Autodesk Fusion 360 part; units mm, degrees
note: some values were not read from the file. Set by a fixed rule: which sketch regions a step uses.
(part 2 of 4)
  spline S338 degree 3 poles (2.6737, -46.2166) (0.624, -45.5094) (-0.7902, -43.8549) (-1.106, -41.9528) (-1.287, -40.8624) (-1.1003, -39.6959) (-0.5192, -38.6497) knots 0 0 0 0 0.618555 0.618555 0.618555 0.973163 0.973163 0.973163 0.973163
  spline S339 degree 3 poles (-0.5192, -38.6497) (-0.9554, -37.9197) (-1.2418, -37.1573) (-1.2576, -36.3503) (-1.2716, -35.6348) (-1.0747, -34.9439) (-0.7598, -34.2709) knots 0.006673 0.006673 0.006673 0.006673 0.533212 0.533212 0.533212 1 1 1 1
  spline S340 degree 3 poles (-0.7598, -34.2709) (0.1145, -32.4027) (1.9335, -31.179) (4.0147, -30.9406) knots 0 0 0 0 0.893312 0.893312 0.893312 0.893312
  spline S341 degree 3 poles (4.0147, -30.9406) (3.9761, -30.3012) (3.9008, -29.105) (3.8396, -28.1591) knots 0.081568 0.081568 0.081568 0.081568 1 1 1 1
  spline S342 degree 3 poles (3.8396, -28.1591) (3.6928, -25.8896) (3.7601, -22.8302) (4.0082, -20.7539) knots 0 0 0 0 1 1 1 1
  spline S343 degree 3 poles (4.0082, -20.7539) (4.7062, -14.9126) (7.125, -9.921) (11.1287, -6.1499) knots 0 0 0 0 1 1 1 1
  constraint coincident L48.end L50
  constraint coincident L49.start S307
  constraint coincident L49.end S308
extrude "Extrude1" add sketch "Sketch1" against normal blind 2 contours S0 L0 L1 S1 S2 L2 L3 S3 S4 S5 S6 S7 S8 S9 S10 S11 S12 S13 S14 S15 S16 L4 L5 S17 S18 S19 L6 L7 S20 S21 S22 S23 S24 S25 L8 L9 S26 S27 L10 L11 S28 S29 S30 S31 S32 S33 S34 S35 S36 S37 S38 S39 S40 L12 L13 S41 S42 S43 S44 S45 S150 L24 L25 S151 S152 L26 L27 S153 S154 S155 S156 S157 S158 S159 S160 S161 S162 S163 S164 S165 S166 L28 L29 S167 S168 S169 L30 L31 S170 S171 S172 S173 S174 S175 L32 L33 S176 S177 L34 L35 S178 S179 S180 S181 S182 S183 S184 S185 S186 S187 S188 S189 S190 L36 L37 S191 S192 S193 S194 S195 | S46 S47 S48 S49 S50 S51 S52 S53 S54 S55 S56 S57 S58 S59 S60 S61 S62 S63 L14 L15 S64 S65 S66 S67 S68 S69 S70 S71 S72 S73 S74 S75 S76 S77 S196 S197 S198 S199 S200 S201 S202 S203 S204 S205 S206 S207 S208 S209 S210 S211 S212 S213 L38 L39 S214 S215 S216 S217 S218 S219 S220 S221 S222 S223 S224 S225 S226 S227 | S78 S79 S80 S81 S82 S83 S84 S85 S86 S87 S88 S89 S90 S91 S92 S93 S94 S95 S96 S97 S98 S99 S100 S101 S102 S103 S104 S105 S106 S107 S228 S229 S230 S231 S232 S233 S234 S235 S236 S237 S238 S239 S240 S241 S242 S243 S244 S245 S246 S247 S248 S249 S250 S251 S252 S253 S254 S255 S256 S257 | S108 S109 S110 S111 S112 S113 S114 S115 S116 L16 L17 S117 S118 S119 L18 L19 S120 S121 S122 S123 S124 S125 S126 S127 S128 S129 S130 S258 S259 S260 S261 S262 S263 S264 S265 S266 L40 L41 S267 S268 S269 L42 L43 S270 S271 S272 S273 S274 S275 S276 S277 S278 S279 S280 | S131 S132 S133 S134 S135 S136 S137 S138 S139 S140 S141 L20 L21 S142 S143 S144 S145 S146 L22 L23 S147 S148 S149 S281 S282 S283 S284 S285 S286 S287 S288 S289 S290 S291 L44 L45 S292 S293 S294 S295 S296 L46 L47 S297 S298 S299 | L49 S300 S301 S302 S303 S304 S305 S306 S307 S308 L50 L51 S309 S310 S311 S312 S313 L52 S314 S315 L53 L54 S316 S317 S318 S319 S320 S321 S322 S323 S324 S325 S326 S327 S328 S329 S330 S331 L55 S332 S333 S334 S335 S336 S337 S338 S339 S340 S341 S342 S343 makes body 1
extrude "Extrude2" add sketch "Sketch1" along normal blind 5 contours S46 S47 S48 S49 S50 S51 S52 S53 S54 S55 S56 S57 S58 S59 S60 S61 S62 S63 L14 L15 S64 S65 S66 S67 S68 S69 S70 S71 S72 S73 S74 S75 S76 S77 S196 S197 S198 S199 S200 S201 S202 S203 S204 S205 S206 S207 S208 S209 S210 S211 S212 S213 L38 L39 S214 S215 S216 S217 S218 S219 S220 S221 S222 S223 S224 S225 S226 S227 | S78 S79 S80 S81 S82 S83 S84 S85 S86 S87 S88 S89 S90 S91 S92 S93 S94 S95 S96 S97 S98 S99 S100 S101 S102 S103 S104 S105 S106 S107 S228 S229 S230 S231 S232 S233 S234 S235 S236 S237 S238 S239 S240 S241 S242 S243 S244 S245 S246 S247 S248 S249 S250 S251 S252 S253 S254 S255 S256 S257 | S108 S109 S110 S111 S112 S113 S114 S115 S116 L16 L17 S117 S118 S119 L18 L19 S120 S121 S122 S123 S124 S125 S126 S127 S128 S129 S130 S258 S259 S260 S261 S262 S263 S264 S265 S266 L40 L41 S267 S268 S269 L42 L43 S270 S271 S272 S273 S274 S275 S276 S277 S278 S279 S280 | S131 S132 S133 S134 S135 S136 S137 S138 S139 S140 S141 L20 L21 S142 S143 S144 S145 S146 L22 L23 S147 S148 S149 S281 S282 S283 S284 S285 S286 S287 S288 S289 S290 S291 L44 L45 S292 S293 S294 S295 S296 L46 L47 S297 S298 S299 bodies 1
extrude "Extrude3" add sketch "Sketch1" along normal blind 10 contours L49 S300 S301 S302 S303 S304 S305 S306 S307 S308 L50 L51 S309 S310 S311 S312 S313 L52 S314 S315 L53 L54 S316 S317 S318 S319 S320 S321 S322 S323 S324 S325 S326 S327 S328 S329 S330 S331 L55 S332 S333 S334 S335 S336 S337 S338 S339 S340 S341 S342 S343 bodies 1
extrude "Extrude4" add sketch "Sketch1" against normal blind 2 separate body contours S0 L0 L1 S1 S2 L2 L3 S3 S4 S5 S6 S7 S8 S9 S10 S11 S12 S13 S14 S15 S16 L4 L5 S17 S18 S19 L6 L7 S20 S21 S22 S23 S24 S25 L8 L9 S26 S27 L10 L11 S28 S29 S30 S31 S32 S33 S34 S35 S36 S37 S38 S39 S40 L12 L13 S41 S42 S43 S44 S45 S150 L24 L25 S151 S152 L26 L27 S153 S154 S155 S156 S157 S158 S159 S160 S161 S162 S163 S164 S165 S166 L28 L29 S167 S168 S169 L30 L31 S170 S171 S172 S173 S174 S175 L32 L33 S176 S177 L34 L35 S178 S179 S180 S181 S182 S183 S184 S185 S186 S187 S188 S189 S190 L36 L37 S191 S192 S193 S194 S195 | L49 S300 S301 S302 S303 S304 S305 S306 S307 S308 L50 L51 S309 S310 S311 S312 S313 L52 S314 S315 L53 L54 S316 S317 S318 S319 S320 S321 S322 S323 S324 S325 S326 S327 S328 S329 S330 S331 L55 S332 S333 S334 S335 S336 S337 S338 S339 S340 S341 S342 S343 makes body 2
extrude "Extrude5" add sketch "Sketch1" along normal blind 5 separate body contours S0 L0 L1 S1 S2 L2 L3 S3 S4 S5 S6 S7 S8 S9 S10 S11 S12 S13 S14 S15 S16 L4 L5 S17 S18 S19 L6 L7 S20 S21 S22 S23 S24 S25 L8 L9 S26 S27 L10 L11 S28 S29 S30 S31 S32 S33 S34 S35 S36 S37 S38 S39 S40 L12 L13 S41 S42 S43 S44 S45 S150 L24 L25 S151 S152 L26 L27 S153 S154 S155 S156 S157 S158 S159 S160 S161 S162 S163 S164 S165 S166 L28 L29 S167 S168 S169 L30 L31 S170 S171 S172 S173 S174 S175 L32 L33 S176 S177 L34 L35 S178 S179 S180 S181 S182 S183 S184 S185 S186 S187 S188 S189 S190 L36 L37 S191 S192 S193 S194 S195 makes body 3
extrude "Extrude6" add sketch "Sketch1" along normal blind 10 contours L49 S300 S301 S302 S303 S304 S305 S306 S307 S308 L50 L51 S309 S310 S311 S312 S313 L52 S314 S315 L53 L54 S316 S317 S318 S319 S320 S321 S322 S323 S324 S325 S326 S327 S328 S329 S330 S331 L55 S332 S333 S334 S335 S336 S337 S338 S339 S340 S341 S342 S343 bodies 2 3
sketch "Sketch2" plane through (0, 0, -2) normal (0, 0, -1) x (1, 0, 0)
  spline S0 degree 3 poles (3.3605, 43.321) (4.2972, 43.7123) (5.127, 43.7031) (6.3837, 43.2874) knots 0 0 0 0 1 1 1 1
  spline S1 degree 3 poles (6.3837, 43.2874) (7.3845, 42.9564) (8.1509, 42.4223) (9.1149, 41.384) knots 0 0 0 0 1 1 1 1
  spline S2 degree 3 poles (9.1149, 41.384) (9.6604, 40.7965) (9.9744, 40.5375) (10.1414, 40.5375) knots 0 0 0 0 1 1 1 1
  spline S3 degree 3 poles (10.1414, 40.5375) (10.2736, 40.5375) (10.8079, 40.801) (11.3285, 41.1231) knots 0 0 0 0 1 1 1 1
  spline S4 degree 3 poles (11.3285, 41.1231) (12.8148, 42.0424) (13.5925, 42.3956) (14.4099, 42.5224) knots 0 0 0 0 1 1 1 1
  spline S5 degree 3 poles (14.4099, 42.5224) (15.7434, 42.7294) (16.8719, 42.2963) (17.2889, 41.4175) knots 0 0 0 0 1 1 1 1
  spline S6 degree 3 poles (17.2889, 41.4175) (17.4425, 41.0937) (17.464, 40.8751) (17.4081, 40.2046) knots 0 0 0 0 1 1 1 1
  spline S7 degree 3 poles (17.4081, 40.2046) (17.3434, 39.4284) (17.3531, 39.3735) (17.5983, 39.1282) knots 0 0 0 0 1 1 1 1
  spline S8 degree 3 poles (17.5983, 39.1282) (17.8995, 38.827) (18.0838, 38.8152) (19.1861, 39.0261) knots 0 0 0 0 1 1 1 1
  spline S9 degree 3 poles (19.1861, 39.0261) (21.2987, 39.4304) (22.4511, 38.9297) (22.4522, 37.607) knots 0 0 0 0 1 1 1 1
  spline S10 degree 3 poles (22.4522, 37.607) (22.4529, 36.7454) (21.8377, 36.2639) (20.7361, 36.2639) knots 0 0 0 0 1 1 1 1
  spline S11 degree 3 poles (20.7361, 36.2639) (20.0382, 36.2639) (19.7425, 36.0347) (19.7425, 35.4937) knots 0 0 0 0 1 1 1 1
  spline S12 degree 3 poles (19.7425, 35.4937) (19.7425, 34.9001) (19.9962, 34.7075) (21.0588, 34.4943) knots 0 0 0 0 1 1 1 1
  spline S13 degree 3 poles (21.0588, 34.4943) (22.1331, 34.2788) (22.5478, 34.0955) (22.8603, 33.6982) knots 0 0 0 0 1 1 1 1
  spline S14 degree 3 poles (22.8603, 33.6982) (23.5958, 32.7632) (22.5543, 31.8861) (20.7083, 31.8861) knots 0 0 0 0 1 1 1 1
  spline S15 degree 3 poles (20.7083, 31.8861) (18.9346, 31.8861) (17.432, 32.5128) (15.9552, 33.8684) knots 0 0 0 0 1 1 1 1
  spline S16 degree 3 poles (15.9552, 33.8684) (15.4567, 34.326) (14.9608, 34.7004) (14.8533, 34.7004) knots 0 0 0 0 1 1 1 1
  spline S17 degree 3 poles (14.8533, 34.7004) (14.7458, 34.7004) (14.4299, 34.5351) (14.1513, 34.333) knots 0 0 0 0 1 1 1 1
  spline S18 degree 3 poles (14.1513, 34.333) (13.8727, 34.1309) (13.3868, 33.8381) (13.0715, 33.6822) knots 0 0 0 0 1 1 1 1
  spline S19 degree 3 poles (13.0715, 33.6822) (11.8711, 33.0889) (10.2509, 33.3985) (9.352, 34.393) knots 0 0 0 0 1 1 1 1
  spline S20 degree 3 poles (9.352, 34.393) (8.4004, 35.4459) (8.1864, 35.6385) (7.9683, 35.6385) knots 0 0 0 0 1 1 1 1
  spline S21 degree 3 poles (7.9683, 35.6385) (7.7171, 35.6385) (7.2977, 35.2383) (6.9738, 34.6891) knots 0 0 0 0 1 1 1 1
  spline S22 degree 3 poles (6.9738, 34.6891) (6.4989, 33.8843) (4.3788, 33.6094) (3.2207, 34.2025) knots 0 0 0 0 1 1 1 1
  spline S23 degree 3 poles (3.2207, 34.2025) (1.9483, 34.8542) (1.3752, 36.0623) (1.9202, 36.9441) knots 0 0 0 0 1 1 1 1
  spline S24 degree 3 poles (1.9202, 36.9441) (2.1572, 37.3277) (2.6853, 37.619) (3.1435, 37.619) knots 0 0 0 0 1 1 1 1
  spline S25 degree 3 poles (3.1435, 37.619) (3.8871, 37.619) (4.3159, 37.943) (4.3159, 38.505) knots 0 0 0 0 1 1 1 1
  spline S26 degree 3 poles (4.3159, 38.505) (4.3159, 39.0685) (4.1681, 39.1932) (3.1927, 39.4522) knots 0 0 0 0 1 1 1 1
  spline S27 degree 3 poles (3.1927, 39.4522) (2.8902, 39.5325) (2.529, 39.6727) (2.39, 39.7638) knots 0 0 0 0 1 1 1 1
  spline S28 degree 3 poles (2.39, 39.7638) (2.0795, 39.9672) (1.7097, 40.7046) (1.7111, 41.1177) knots 0 0 0 0 1 1 1 1
  spline S29 degree 3 poles (1.7111, 41.1177) (1.7137, 41.8847) (2.5286, 42.9734) (3.3605, 43.321) knots 0 0 0 0 1 1 1 1
  spline S30 degree 3 poles (8.0031, 33.0312) (8.0532, 33.032) (8.369, 32.8492) (8.705, 32.6248) knots 0 0 0 0 1 1 1 1
  spline S31 degree 3 poles (8.705, 32.6248) (9.2851, 32.2374) (9.8665, 32.0076) (11.2214, 31.6303) knots 0 0 0 0 1 1 1 1
  spline S32 degree 3 poles (11.2214, 31.6303) (11.8742, 31.4485) (11.8914, 31.4155) (11.7143, 30.6874) knots 0 0 0 0 1 1 1 1
  spline S33 degree 3 poles (11.7143, 30.6874) (10.9845, 27.6875) (10.9096, 23.7891) (11.5242, 20.7853) knots 0 0 0 0 1 1 1 1
  spline S34 degree 3 poles (11.5242, 20.7853) (12.8947, 14.087) (17.7674, 9.0084) (23.8364, 7.9527) knots 0 0 0 0 1 1 1 1
  spline S35 degree 3 poles (23.8364, 7.9527) (24.5674, 7.8255) (25.2101, 7.7982) (26.5177, 7.8388) knots 0 0 0 0 1 1 1 1
  spline S36 degree 3 poles (26.5177, 7.8388) (28.4619, 7.8992) (29.3901, 8.1006) (31.078, 8.8283) knots 0 0 0 0 1 1 1 1
  spline S37 degree 3 poles (31.078, 8.8283) (35.3425, 10.6668) (38.7599, 15.2726) (39.9599, 20.7989) knots 0 0 0 0 1 1 1 1
  spline S38 degree 3 poles (39.9599, 20.7989) (40.381, 22.7381) (40.5138, 24.5489) (40.4444, 27.4041) knots 0 0 0 0 1 1 1 1
  spline S39 degree 3 poles (40.4444, 27.4041) (40.4089, 28.866) (40.3511, 30.4904) (40.316, 31.014) knots 0 0 0 0 1 1 1 1
  line L0 (40.316, 31.014) -> (40.2522, 31.966)
  line L1 (40.2522, 31.966) -> (41.7662, 32.4472)
  spline S40 degree 3 poles (41.7662, 32.4472) (42.5989, 32.7119) (43.3335, 32.9285) (43.3985, 32.9285) knots 0 0 0 0 1 1 1 1
  spline S41 degree 3 poles (43.3985, 32.9285) (43.4636, 32.9285) (43.808, 32.6862) (44.1638, 32.39) knots 0 0 0 0 1 1 1 1
  spline S42 degree 3 poles (44.1638, 32.39) (44.5196, 32.0939) (45.2044, 31.6627) (45.6856, 31.4317) knots 0 0 0 0 1 1 1 1
  line L2 (45.6856, 31.4317) -> (46.5605, 31.0119)
  line L3 (46.5605, 31.0119) -> (46.4885, 28.8171)
  spline S43 degree 3 poles (46.4885, 28.8171) (46.2828, 22.5508) (45.6972, 17.9425) (44.4939, 13.1206) knots 0 0 0 0 1 1 1 1
  spline S44 degree 3 poles (44.4939, 13.1206) (43.6086, 9.573) (42.6843, 7.6473) (41.0419, 5.9282) knots 0 0 0 0 1 1 1 1
  spline S45 degree 3 poles (41.0419, 5.9282) (39.2602, 4.0633) (36.9993, 2.991) (33.5472, 2.3735) knots 0 0 0 0 1 1 1 1
  spline S46 degree 3 poles (33.5472, 2.3735) (32.3588, 2.1609) (31.8638, 2.1321) (29.3841, 2.1308) knots 0 0 0 0 1 1 1 1
  spline S47 degree 3 poles (29.3841, 2.1308) (26.2893, 2.1292) (25.7344, 2.1938) (23.1155, 2.861) knots 0 0 0 0 1 1 1 1
  spline S48 degree 3 poles (23.1155, 2.861) (15.8271, 4.7179) (10.0738, 9.8891) (7.9282, 16.5117) knots 0 0 0 0 1 1 1 1
  spline S49 degree 3 poles (7.9282, 16.5117) (7.4178, 18.087) (7.2808, 18.6726) (7.0133, 20.4204) knots 0 0 0 0 1 1 1 1
  spline S50 degree 3 poles (7.0133, 20.4204) (6.814, 21.7234) (6.7809, 22.3775) (6.7737, 25.1631) knots 0 0 0 0 1 1 1 1
  spline S51 degree 3 poles (6.7737, 25.1631) (6.7643, 28.8189) (6.9545, 31.8997) (7.2227, 32.4341) knots 0 0 0 0 1 1 1 1
  spline S52 degree 3 poles (7.2227, 32.4341) (7.3731, 32.7338) (7.7563, 33.027) (8.0031, 33.0312) knots 0 0 0 0 1 1 1 1
  spline S53 degree 3 poles (36.8022, 32.72) (36.8147, 32.72) (37.1676, 32.5951) (37.5865, 32.4424) knots 0 0 0 0 1 1 1 1
  spline S54 degree 3 poles (37.5865, 32.4424) (38.0054, 32.2897) (38.358, 32.1588) (38.3699, 32.1514) knots 0 0 0 0 1 1 1 1
  spline S55 degree 3 poles (38.3699, 32.1514) (38.3819, 32.1441) (38.4663, 31.4364) (38.5576, 30.5789) knots 0 0 0 0 1 1 1 1
  spline S56 degree 3 poles (38.5576, 30.5789) (38.7576, 28.7005) (38.787, 24.9492) (38.613, 23.4953) knots 0 0 0 0 1 1 1 1
  spline S57 degree 3 poles (38.613, 23.4953) (38.0797, 19.0373) (36.5859, 15.601) (34.0858, 13.0806) knots 0 0 0 0 1 1 1 1
  spline S58 degree 3 poles (34.0858, 13.0806) (32.465, 11.4468) (30.6163, 10.3222) (28.7127, 9.8123) knots 0 0 0 0 1 1 1 1
  spline S59 degree 3 poles (28.7127, 9.8123) (27.353, 9.4481) (25.087, 9.4274) (23.6217, 9.7658) knots 0 0 0 0 1 1 1 1
  spline S60 degree 3 poles (23.6217, 9.7658) (21.0994, 10.3485) (19.0072, 11.5487) (17.1769, 13.463) knots 0 0 0 0 1 1 1 1
  spline S61 degree 3 poles (17.1769, 13.463) (13.6018, 17.2023) (12.102, 22.8928) (13.1278, 28.8262) knots 0 0 0 0 1 1 1 1
  spline S62 degree 3 poles (13.1278, 28.8262) (13.3528, 30.1278) (13.671, 31.4351) (13.8593, 31.832) knots 0 0 0 0 1 1 1 1
  spline S63 degree 3 poles (13.8593, 31.832) (14.0085, 32.1465) (14.374, 32.4073) (14.6654, 32.4073) knots 0 0 0 0 1 1 1 1
  spline S64 degree 3 poles (14.6654, 32.4073) (14.734, 32.4073) (15.313, 32.0502) (15.9519, 31.6138) knots 0 0 0 0 1 1 1 1
  line L4 (15.9519, 31.6138) -> (17.1137, 30.8202)
  line L5 (17.1137, 30.8202) -> (17.1634, 28.2522)
  spline S65 degree 3 poles (17.1634, 28.2522) (17.2317, 24.7162) (17.5594, 23.0905) (18.6473, 20.8895) knots 0 0 0 0 1 1 1 1
  spline S66 degree 3 poles (18.6473, 20.8895) (19.9291, 18.2961) (21.9531, 16.557) (24.3463, 15.9928) knots 0 0 0 0 1 1 1 1
  spline S67 degree 3 poles (24.3463, 15.9928) (25.1987, 15.7919) (26.7215, 15.7913) (27.512, 15.9915) knots 0 0 0 0 1 1 1 1
  spline S68 degree 3 poles (27.512, 15.9915) (30.0811, 16.6424) (32.4074, 19.0232) (33.3899, 22.0071) knots 0 0 0 0 1 1 1 1
  spline S69 degree 3 poles (33.3899, 22.0071) (33.9317, 23.6526) (34.039, 24.4827) (34.0972, 27.4794) knots 0 0 0 0 1 1 1 1
  line L6 (34.0972, 27.4794) -> (34.1523, 30.317)
  line L7 (34.1523, 30.317) -> (34.6867, 30.7314)
  spline S70 degree 3 poles (34.6867, 30.7314) (34.9807, 30.9594) (35.5718, 31.5) (36.0003, 31.9329) knots 0 0 0 0 1 1 1 1
  spline S71 degree 3 poles (36.0003, 31.9329) (36.4288, 32.3658) (36.7897, 32.72) (36.8022, 32.72) knots 0 0 0 0 1 1 1 1
  spline S72 degree 3 poles (40.3105, 43.3948) (41.3954, 43.901) (42.2636, 43.9539) (43.1464, 43.5675) knots 0 0 0 0 1 1 1 1
  spline S73 degree 3 poles (43.1464, 43.5675) (43.6121, 43.3637) (44.0986, 42.8484) (44.1975, 42.454) knots 0 0 0 0 1 1 1 1
  spline S74 degree 3 poles (44.1975, 42.454) (44.2329, 42.313) (44.2296, 41.9062) (44.1901, 41.55) knots 0 0 0 0 1 1 1 1
  spline S75 degree 3 poles (44.1901, 41.55) (44.0616, 40.3913) (44.0787, 40.2083) (44.3356, 40.0003) knots 0 0 0 0 1 1 1 1
  spline S76 degree 3 poles (44.3356, 40.0003) (44.7112, 39.6961) (45.1086, 39.7683) (46.0893, 40.3188) knots 0 0 0 0 1 1 1 1
  spline S77 degree 3 poles (46.0893, 40.3188) (47.5056, 41.1136) (48.2545, 41.3947) (49.1098, 41.4522) knots 0 0 0 0 1 1 1 1
  spline S78 degree 3 poles (49.1098, 41.4522) (50.0601, 41.5161) (50.6688, 41.3509) (51.2194, 40.8796) knots 0 0 0 0 1 1 1 1
  spline S79 degree 3 poles (51.2194, 40.8796) (51.7463, 40.4286) (51.9622, 40.0221) (51.9699, 39.4669) knots 0 0 0 0 1 1 1 1
  spline S80 degree 3 poles (51.9699, 39.4669) (51.9747, 39.1179) (51.9177, 38.9851) (51.6667, 38.7609) knots 0 0 0 0 1 1 1 1
  spline S81 degree 3 poles (51.6667, 38.7609) (51.4967, 38.6089) (51.1707, 38.4548) (50.9423, 38.4183) knots 0 0 0 0 1 1 1 1
  spline S82 degree 3 poles (50.9423, 38.4183) (50.0539, 38.2762) (49.4995, 37.6121) (49.7804, 37.0264) knots 0 0 0 0 1 1 1 1
  spline S83 degree 3 poles (49.7804, 37.0264) (49.9949, 36.579) (50.335, 36.453) (51.1465, 36.5202) knots 0 0 0 0 1 1 1 1
  spline S84 degree 3 poles (51.1465, 36.5202) (51.7992, 36.5743) (51.8736, 36.5589) (52.1107, 36.3219) knots 0 0 0 0 1 1 1 1
  spline S85 degree 3 poles (52.1107, 36.3219) (52.632, 35.8005) (52.3398, 34.5008) (51.5692, 33.913) knots 0 0 0 0 1 1 1 1
  spline S86 degree 3 poles (51.5692, 33.913) (50.1664, 32.8431) (48.1142, 32.4761) (46.4453, 32.9969) knots 0 0 0 0 1 1 1 1
  spline S87 degree 3 poles (46.4453, 32.9969) (45.8057, 33.1965) (44.9544, 33.904) (44.6602, 34.4802) knots 0 0 0 0 1 1 1 1
  spline S88 degree 3 poles (44.6602, 34.4802) (44.2129, 35.3568) (43.7112, 35.4679) (42.8564, 34.8799) knots 0 0 0 0 1 1 1 1
  spline S89 degree 3 poles (42.8564, 34.8799) (42.5554, 34.6729) (42.0276, 34.3719) (41.6837, 34.2111) knots 0 0 0 0 1 1 1 1
  spline S90 degree 3 poles (41.6837, 34.2111) (41.1075, 33.9417) (40.9598, 33.9187) (39.8075, 33.9187) knots 0 0 0 0 1 1 1 1
  line L8 (39.8075, 33.9187) -> (38.5567, 33.9187)
  line L9 (38.5567, 33.9187) -> (37.6186, 34.4148)
  spline S91 degree 3 poles (37.6186, 34.4148) (37.1026, 34.6877) (36.539, 34.9376) (36.3661, 34.9702) knots 0 0 0 0 1 1 1 1
  spline S92 degree 3 poles (36.3661, 34.9702) (35.922, 35.0539) (35.5337, 34.7143) (35.1462, 33.9031) knots 0 0 0 0 1 1 1 1
  spline S93 degree 3 poles (35.1462, 33.9031) (34.2767, 32.0829) (32.5077, 31.1785) (31.2082, 31.8899) knots 0 0 0 0 1 1 1 1
  spline S94 degree 3 poles (31.2082, 31.8899) (30.5745, 32.2368) (30.2974, 32.7818) (30.4669, 33.3475) knots 0 0 0 0 1 1 1 1
  spline S95 degree 3 poles (30.4669, 33.3475) (30.6161, 33.8457) (31.3598, 34.532) (32.2646, 35.0067) knots 0 0 0 0 1 1 1 1
  spline S96 degree 3 poles (32.2646, 35.0067) (33.1402, 35.466) (33.3971, 35.7096) (33.3971, 36.0805) knots 0 0 0 0 1 1 1 1
  spline S97 degree 3 poles (33.3971, 36.0805) (33.3971, 36.501) (33.238, 36.7542) (32.8468, 36.9565) knots 0 0 0 0 1 1 1 1
  spline S98 degree 3 poles (32.8468, 36.9565) (31.0444, 37.8883) (30.5759, 39.9699) (31.8443, 41.4109) knots 0 0 0 0 1 1 1 1
  spline S99 degree 3 poles (31.8443, 41.4109) (32.3815, 42.0212) (32.9483, 42.3169) (33.7139, 42.3863) knots 0 0 0 0 1 1 1 1
  spline S100 degree 3 poles (33.7139, 42.3863) (34.5937, 42.4661) (35.2523, 42.2098) (36.037, 41.4824) knots 0 0 0 0 1 1 1 1
  spline S101 degree 3 poles (36.037, 41.4824) (36.3909, 41.1543) (36.763, 40.8557) (36.8638, 40.8189) knots 0 0 0 0 1 1 1 1
  spline S102 degree 3 poles (36.8638, 40.8189) (37.192, 40.6989) (37.5089, 40.9167) (38.6147, 42.0227) knots 0 0 0 0 1 1 1 1
  spline S103 degree 3 poles (38.6147, 42.0227) (39.4081, 42.8162) (39.8679, 43.1882) (40.3105, 43.3948) knots 0 0 0 0 1 1 1 1
  spline S104 degree 3 poles (3.8396, 28.1591) (3.6928, 25.8896) (3.7601, 22.8302) (4.0082, 20.7539) knots 0 0 0 0 1 1 1 1
  ellipse E0 centre (58.4946, 46.0269) end of major axis (108.5558, 82.8636) minor radius 37.1858 (4.0082, 20.7539) -> (11.1287, 6.1499) ccw
  spline S105 degree 3 poles (11.1287, 6.1499) (15.8219, 1.7292) (21.8181, -0.6374) (28.7719, -0.8627) knots 0 0 0 0 1 1 1 1
  ellipse E1 centre (5.0131, 40.0097) end of major axis (43.6862, 4.3261) minor radius 27.1643 (28.7719, -0.8627) -> (39.0808, 0.9877) ccw
  spline S106 degree 3 poles (39.0808, 0.9877) (40.5743, 1.6901) (41.6727, 2.4153) (42.7258, 3.4112) knots 0 0 0 0 1 1 1 1
  spline S107 degree 3 poles (42.7258, 3.4112) (44.4016, 4.9959) (45.589, 6.8874) (46.5056, 9.5421) (46.9414, 10.8042) (47.3249, 12.2429) (47.6965, 13.9335) knots 0 0 0 0 0.677783 0.677783 0.677783 1 1 1 1
  spline S108 degree 3 poles (47.6965, 13.9335) (48.7263, 18.6186) (49.1132, 21.8227) (49.3958, 27.9744) knots 0 0 0 0 1 1 1 1
  ellipse E2 centre (49.445, 28.2243) end of major axis (49.5599, 30.6408) minor radius 0.0375 (49.4993, 29.9265) -> (49.3958, 27.9744) ccw
  spline S109 degree 3 poles (49.4993, 29.9265) (51.3935, 30.3328) (52.9435, 31.0564) (54.0116, 32.193) (54.363, 32.5669) (54.6579, 32.9856) (54.882, 33.4409) knots 0.033409 0.033409 0.033409 0.033409 0.760746 0.760746 0.760746 0.999997 0.999997 0.999997 0.999997
  spline S110 degree 3 poles (54.882, 33.4409) (55.0347, 33.7513) (55.1727, 34.0995) (55.2323, 34.4752) (55.2709, 34.7187) (55.2821, 34.9498) (55.2846, 35.2136) knots 0 0 0 0 0.549059 0.549059 0.549059 0.90483 0.90483 0.90483 0.90483
  line L10 (55.2846, 35.2136) -> (55.2832, 35.6451)
  spline S111 degree 3 poles (55.2832, 35.6451) (55.2771, 35.9972) (55.2543, 36.309) (55.1786, 36.6345) (55.1024, 36.9617) (54.9878, 37.2507) (54.8436, 37.5871) knots 0.088946 0.088946 0.088946 0.088946 0.543269 0.543269 0.543269 1 1 1 1
  line L11 (54.8436, 37.5871) -> (54.6708, 37.9902)
  line L12 (54.6708, 37.9902) -> (54.7256, 38.1789)
  spline S112 degree 3 poles (54.7256, 38.1789) (55.1949, 39.793) (54.7298, 41.4712) (53.6604, 42.6498) (52.9721, 43.4084) (52.0402, 43.976) (50.9574, 44.2653) knots 0 0 0 0 0.608426 0.608426 0.608426 1 1 1 1
  spline S113 degree 3 poles (50.9574, 44.2653) (49.8818, 44.5526) (48.7117, 44.4734) (47.3744, 44.1183) (47.178, 44.0661) (46.9771, 44.0079) (46.771, 43.9438) knots 0 0 0 0 0.824545 0.824545 0.824545 0.945665 0.945665 0.945665 0.945665
  spline S114 degree 3 poles (46.771, 43.9438) (46.7093, 44.062) (46.6405, 44.1796) (46.5676, 44.2944) (46.2623, 44.7749) (45.8902, 45.2321) (45.4363, 45.6075) (45.3884, 45.647) (45.3392, 45.6858) (45.2879, 45.7236) knots 0.223295 0.223295 0.223295 0.223295 0.361232 0.361232 0.361232 0.939053 0.939053 0.939053 1 1 1 1
  spline S115 degree 3 poles (45.2879, 45.7236) (44.2745, 46.4714) (42.9911, 46.772) (41.707, 46.737) (41.2318, 46.724) (40.7551, 46.6601) (40.2904, 46.5351) knots 0.000002 0.000002 0.000002 0.000002 0.729882 0.729882 0.729882 1 1 1 1
  spline S116 degree 3 poles (40.2904, 46.5351) (39.1403, 46.2258) (38.0053, 45.5417) (37.0282, 44.651) knots 0.000001 0.000001 0.000001 0.000001 1 1 1 1
  line L13 (37.0282, 44.651) -> (36.9035, 44.5374)
  spline S117 degree 3 poles (36.9035, 44.5374) (35.1678, 45.5188) (33.1775, 45.6076) (31.5191, 44.8193) (30.4628, 44.3172) (29.5504, 43.4745) (28.8905, 42.373) knots 0.019099 0.019099 0.019099 0.019099 0.618328 0.618328 0.618328 1 1 1 1
  spline S118 degree 3 poles (28.8905, 42.373) (28.2356, 41.2799) (28.0251, 39.987) (28.2891, 38.7134) (28.4327, 38.0204) (28.7011, 37.3303) (29.0737, 36.6286) knots 0 0 0 0 0.647645 0.647645 0.647645 1 1 1 1
  line L14 (29.0737, 36.6286) -> (29.1612, 36.4638)
  line L15 (29.1612, 36.4638) -> (28.9908, 36.2914)
  spline S119 degree 3 poles (28.9908, 36.2914) (28.3897, 35.6836) (27.931, 35.0843) (27.6841, 34.3672) (27.522, 33.8963) (27.4651, 33.4076) (27.4689, 32.9193) knots 0 0 0 0 0.603605 0.603605 0.603605 1 1 1 1
  spline S120 degree 3 poles (27.4689, 32.9193) (27.4781, 31.7149) (28.0681, 30.6219) (28.9533, 29.8689) (29.5522, 29.3594) (30.2878, 28.9905) (31.1058, 28.7908) knots 0 0 0 0 0.569109 0.569109 0.569109 0.954182 0.954182 0.954182 0.954182
  ellipse E3 centre (31.0764, 27.6801) end of major axis (31.0429, 29.675) minor radius 0.0578 (31.1352, 27.6181) -> (31.1058, 28.7908) ccw
  spline S121 degree 3 poles (31.1352, 27.6181) (31.1644, 25.7831) (31.0814, 24.7731) (30.8193, 23.7418) (30.754, 23.485) (30.6766, 23.2243) (30.5839, 22.9462) knots 0 0 0 0 0.800641 0.800641 0.800641 1 1 1 1
  spline S122 degree 3 poles (30.5839, 22.9462) (29.9756, 21.1214) (28.9014, 19.8352) (27.6291, 19.2047) knots 0 0 0 0 1 1 1 1
  spline S123 degree 3 poles (27.6291, 19.2047) (26.8945, 18.8407) (26.4461, 18.7298) (25.9454, 18.7349) (25.7421, 18.7369) (25.5228, 18.7611) (25.2651, 18.8137) knots 0 0 0 0 0.711303 0.711303 0.711303 1 1 1 1
  spline S124 degree 3 poles (25.2651, 18.8137) (23.7232, 19.1281) (22.4595, 20.0877) (21.5265, 21.709) (21.0344, 22.5641) (20.647, 23.6026) (20.4034, 24.8024) knots 0 0 0 0 0.654705 0.654705 0.654705 1 1 1 1
  spline S125 degree 3 poles (20.4034, 24.8024) (20.2739, 25.4408) (20.1421, 26.5799) (20.0696, 27.6039) (20.0342, 28.1041) (20.0114, 28.5828) (20.0045, 28.9687) knots 0 0 0 0 0.457255 0.457255 0.457255 0.680586 0.680586 0.680586 0.680586
  ellipse E4 centre (21.8994, 28.801) end of major axis (24.7102, 28.7135) minor radius 0.1473 (20.5728, 28.9721) -> (20.0045, 28.9687) ccw
  spline S126 degree 3 poles (20.5728, 28.9721) (21.4581, 28.9695) (21.9205, 28.9661) (22.3941, 29.0471) (22.71, 29.1012) (22.9935, 29.2034) (23.2325, 29.3044) knots 0 0 0 0 0.599835 0.599835 0.599835 1 1 1 1
  spline S127 degree 3 poles (23.2325, 29.3044) (24.2399, 29.7303) (25.0756, 30.3613) (25.5649, 31.2416) (25.8255, 31.7103) (25.9766, 32.236) (26.0196, 32.7724) knots 0.000002 0.000002 0.000002 0.000002 0.65253 0.65253 0.65253 1 1 1 1
  spline S128 degree 3 poles (26.0196, 32.7724) (26.0464, 33.1056) (26.0575, 33.4303) (25.9898, 33.7774) (25.9304, 34.0819) (25.8237, 34.343) (25.7057, 34.6008) knots 0 0 0 0 0.532706 0.532706 0.532706 1 1 1 1
  ellipse E5 centre (16.0287, 33.8196) end of major axis (26.0555, 32.469) minor radius 5.942 (25.7057, 34.6008) -> (25.0063, 35.7274) ccw
  spline S129 degree 3 poles (25.0063, 35.7274) (25.2152, 36.1653) (25.3445, 36.6528) (25.3876, 37.161) (25.3966, 37.268) (25.4033, 37.3773) (25.4085, 37.4918) knots 0.077995 0.077995 0.077995 0.077995 0.83962 0.83962 0.83962 1 1 1 1
  spline S130 degree 3 poles (25.4085, 37.4918) (25.4258, 37.868) (25.439, 38.1756) (25.3733, 38.5347) (25.3129, 38.8652) (25.1915, 39.151) (25.0593, 39.4265) (25.0387, 39.4695) (25.0174, 39.513) (24.9954, 39.5579) knots 0 0 0 0 0.484601 0.484601 0.484601 0.930484 0.930484 0.930484 1 1 1 1
  spline S131 degree 3 poles (24.9954, 39.5579) (24.5918, 40.3776) (23.9772, 41.085) (23.1648, 41.5103) (22.385, 41.9186) (21.4967, 42.0784) (20.4603, 42.1269) knots 0 0 0 0 0.510228 0.510228 0.510228 1 1 1 1
  line L16 (20.4603, 42.1269) -> (20.1789, 42.1401)
  spline S132 degree 3 poles (20.1789, 42.1401) (19.8683, 42.9655) (19.3311, 43.6836) (18.669, 44.2614) (18.1917, 44.6778) (17.6457, 45.021) (17.0294, 45.2285) knots 0.1236 0.1236 0.1236 0.1236 0.632884 0.632884 0.632884 1 1 1 1
  spline S133 degree 3 poles (17.0294, 45.2285) (15.6679, 45.6868) (14.1945, 45.6326) (12.6935, 45.1125) (12.1298, 44.9172) (11.5566, 44.6602) (10.9624, 44.3448) knots 0 0 0 0 0.726997 0.726997 0.726997 1 1 1 1
  spline S134 degree 3 poles (10.9624, 44.3448) (10.8083, 44.263) (10.6793, 44.1929) (10.573, 44.1362) knots 0 0 0 0 0.122244 0.122244 0.122244 0.122244
  spline S135 degree 3 poles (10.573, 44.1362) (10.4946, 44.2052) (10.4022, 44.2872) (10.2936, 44.382) knots 0.893888 0.893888 0.893888 0.893888 1 1 1 1
  ellipse E6 centre (-1.4228, 24.3555) end of major axis (-10.8734, 2.8827) minor radius 14.2538 (10.2936, 44.382) -> (7.2449, 46.1286) ccw
  spline S136 degree 3 poles (7.2449, 46.1286) (6.4114, 46.403) (5.4613, 46.5014) (4.5483, 46.4889) (3.8849, 46.4798) (3.2641, 46.4203) (2.6738, 46.2166) knots 0.000001 0.000001 0.000001 0.000001 0.579134 0.579134 0.579134 1 1 1 1
  spline S137 degree 3 poles (2.6737, 46.2166) (0.624, 45.5094) (-0.7902, 43.8549) (-1.106, 41.9528) (-1.287, 40.8624) (-1.1003, 39.6959) (-0.5192, 38.6497) knots 0 0 0 0 0.618555 0.618555 0.618555 0.973163 0.973163 0.973163 0.973163
  spline S138 degree 3 poles (-0.5192, 38.6497) (-0.9554, 37.9197) (-1.2418, 37.1573) (-1.2576, 36.3503) (-1.2716, 35.6348) (-1.0747, 34.9439) (-0.7598, 34.2709) knots 0.006673 0.006673 0.006673 0.006673 0.533212 0.533212 0.533212 1 1 1 1
  spline S139 degree 3 poles (-0.7598, 34.2709) (0.1145, 32.4027) (1.9335, 31.179) (4.0147, 30.9406) knots 0 0 0 0 0.893312 0.893312 0.893312 0.893312
  spline S140 degree 3 poles (4.0147, 30.9406) (3.9761, 30.3012) (3.9008, 29.105) (3.8396, 28.1591) knots 0.081568 0.081568 0.081568 0.081568 1 1 1 1
  spline S141 degree 5 poles (28.0734, 16.1624) (28.0438, 15.2899) (28.0307, 13.6256) (28.1495, 11.3704) (28.5582, 8.789) (29.4292, 6.1002) (30.4239, 4.31) (31.3732, 3.1762) (32.107, 2.5202) (32.4991, 2.2173) knots 0 0 0 0 0 0 0.2 0.4 0.6 0.8 1 1 1 1 1 1
  line L17 (31.5808, 2.9267) -> (33.4174, 1.5078)
  line L18 (28.1469, 18.3247) -> (28, 14)
  spline S142 degree 3 poles (26.0746, 16.2303) (25.9428, 12.349) (26.3323, 9.3028) (27.1887, 6.732) (27.8662, 4.6985) (28.8531, 2.92) (30.2998, 1.489) (30.6064, 1.1859) (30.9326, 0.9002) (31.2764, 0.6346) knots 0 0 0 0 0.510571 0.510571 0.510571 0.914429 0.914429 0.914429 1 1 1 1
  dimension "d20" = 2
  constraint coincident S68 S141.start
  constraint coincident S46 S141.end
  constraint midpoint S141.end L17
  constraint midpoint S141.start L18
extrude "Extrude7" add sketch "Sketch2" against normal blind 2 separate body contours S36 S59 S141 S142 | S36 S46 S141 S142 | S59 S67 S68 S141 S142 makes body 4
combine "Combine1" operation add target body 4 tool bodies 2 keep tools
sketch "Sketch3" plane through (0, 0, -2) normal (0, 0, -1) x (1, 0, 0)
  spline S0 degree 3 poles (26.0631, 15.8423) (26.0024, 13.4447) (26.1457, 11.3703) (26.4797, 9.5307) knots 0.017136 0.017136 0.017136 0.017136 0.337125 0.337125 0.337125 0.337125
  spline S1 degree 3 poles (26.4797, 9.5307) (25.4741, 9.5023) (24.427, 9.5799) (23.6217, 9.7658) knots 0.450431 0.450431 0.450431 0.450431 1 1 1 1
  spline S2 degree 3 poles (23.6217, 9.7658) (21.0994, 10.3485) (19.0072, 11.5487) (17.1769, 13.463) knots 0 0 0 0 1 1 1 1
  spline S3 degree 3 poles (17.1769, 13.463) (13.6018, 17.2023) (12.102, 22.8928) (13.1278, 28.8262) knots 0 0 0 0 1 1 1 1
  spline S4 degree 3 poles (13.1278, 28.8262) (13.3528, 30.1278) (13.671, 31.4351) (13.8593, 31.832) knots 0 0 0 0 1 1 1 1
  spline S5 degree 3 poles (13.8593, 31.832) (14.0085, 32.1465) (14.374, 32.4073) (14.6654, 32.4073) knots 0 0 0 0 1 1 1 1
  spline S6 degree 3 poles (14.6654, 32.4073) (14.734, 32.4073) (15.313, 32.0502) (15.9519, 31.6138) knots 0 0 0 0 1 1 1 1
  line L0 (15.9519, 31.6138) -> (17.1137, 30.8202)
  line L1 (17.1137, 30.8202) -> (17.1634, 28.2522)
  spline S7 degree 3 poles (17.1634, 28.2522) (17.2317, 24.7162) (17.5594, 23.0905) (18.6473, 20.8895) knots 0 0 0 0 1 1 1 1
  spline S8 degree 3 poles (18.6473, 20.8895) (19.9291, 18.2961) (21.9531, 16.557) (24.3463, 15.9928) knots 0 0 0 0 1 1 1 1
  spline S9 degree 3 poles (24.3463, 15.9928) (24.7994, 15.886) (25.4418, 15.8358) (26.0631, 15.8423) knots 0 0 0 0 0.531523 0.531523 0.531523 0.531523
  spline S10 degree 5 poles (28.8667, 8.0774) (28.9794, 7.6798) (29.2738, 6.7511) (29.8256, 5.3923) (30.5166, 4.1992) (31.3732, 3.1762) (32.107, 2.5202) (32.4991, 2.2173) knots 0.458614 0.458614 0.458614 0.458614 0.458614 0.458614 0.6 0.8 1 1 1 1 1 1
  spline S11 degree 3 poles (28.8667, 8.0774) (29.5627, 8.226) (30.2228, 8.4596) (31.078, 8.8283) knots 0.493372 0.493372 0.493372 0.493372 1 1 1 1
  spline S12 degree 3 poles (31.078, 8.8283) (35.3425, 10.6668) (38.7599, 15.2726) (39.9599, 20.7989) knots 0 0 0 0 1 1 1 1
  spline S13 degree 3 poles (39.9599, 20.7989) (40.381, 22.7381) (40.5138, 24.5489) (40.4444, 27.4041) knots 0 0 0 0 1 1 1 1
  spline S14 degree 3 poles (40.4444, 27.4041) (40.4089, 28.866) (40.3511, 30.4904) (40.316, 31.014) knots 0 0 0 0 1 1 1 1
  line L2 (40.316, 31.014) -> (40.2522, 31.966)
  line L3 (40.2522, 31.966) -> (41.7662, 32.4472)
  spline S15 degree 3 poles (41.7662, 32.4472) (42.5989, 32.7119) (43.3335, 32.9285) (43.3985, 32.9285) knots 0 0 0 0 1 1 1 1
  spline S16 degree 3 poles (43.3985, 32.9285) (43.4636, 32.9285) (43.808, 32.6862) (44.1638, 32.39) knots 0 0 0 0 1 1 1 1
  spline S17 degree 3 poles (44.1638, 32.39) (44.5196, 32.0939) (45.2044, 31.6627) (45.6856, 31.4317) knots 0 0 0 0 1 1 1 1
  line L4 (45.6856, 31.4317) -> (46.5605, 31.0119)
  line L5 (46.5605, 31.0119) -> (46.4885, 28.8171)
  spline S18 degree 3 poles (46.4885, 28.8171) (46.2828, 22.5508) (45.6972, 17.9425) (44.4939, 13.1206) knots 0 0 0 0 1 1 1 1
  spline S19 degree 3 poles (44.4939, 13.1206) (43.6086, 9.573) (42.6843, 7.6473) (41.0419, 5.9282) knots 0 0 0 0 1 1 1 1
  spline S20 degree 3 poles (41.0419, 5.9282) (39.2602, 4.0633) (36.9993, 2.991) (33.5472, 2.3735) knots 0 0 0 0 1 1 1 1
  spline S21 degree 3 poles (33.5472, 2.3735) (33.1543, 2.3032) (32.8372, 2.253) (32.4991, 2.2173) knots 0 0 0 0 0.330606 0.330606 0.330606 0.330606
  spline S22 degree 3 poles (28.0734, 16.1624) (30.4154, 16.9952) (32.4795, 19.2422) (33.3899, 22.0071) knots 0.073406 0.073406 0.073406 0.073406 1 1 1 1
  spline S23 degree 3 poles (33.3899, 22.0071) (33.9317, 23.6526) (34.039, 24.4827) (34.0972, 27.4794) knots 0 0 0 0 1 1 1 1
  line L6 (34.0972, 27.4794) -> (34.1523, 30.317)
  line L7 (34.1523, 30.317) -> (34.6867, 30.7314)
  spline S24 degree 3 poles (34.6867, 30.7314) (34.9807, 30.9594) (35.5718, 31.5) (36.0003, 31.9329) knots 0 0 0 0 1 1 1 1
  spline S25 degree 3 poles (36.0003, 31.9329) (36.4288, 32.3658) (36.7897, 32.72) (36.8022, 32.72) knots 0 0 0 0 1 1 1 1
  spline S26 degree 3 poles (36.8022, 32.72) (36.8147, 32.72) (37.1676, 32.5951) (37.5865, 32.4424) knots 0 0 0 0 1 1 1 1
  spline S27 degree 3 poles (37.5865, 32.4424) (38.0054, 32.2897) (38.358, 32.1588) (38.3699, 32.1514) knots 0 0 0 0 1 1 1 1
  spline S28 degree 3 poles (38.3699, 32.1514) (38.3819, 32.1441) (38.4663, 31.4364) (38.5576, 30.5789) knots 0 0 0 0 1 1 1 1
  spline S29 degree 3 poles (38.5576, 30.5789) (38.7576, 28.7005) (38.787, 24.9492) (38.613, 23.4953) knots 0 0 0 0 1 1 1 1
  spline S30 degree 3 poles (38.613, 23.4953) (38.0797, 19.0373) (36.5859, 15.601) (34.0858, 13.0806) knots 0 0 0 0 1 1 1 1
  spline S31 degree 3 poles (34.0858, 13.0806) (32.465, 11.4468) (30.6163, 10.3222) (28.7127, 9.8123) knots 0 0 0 0 1 1 1 1
  spline S32 degree 3 poles (28.7127, 9.8123) (28.6362, 9.7918) (28.5569, 9.7724) (28.475, 9.7541) knots 0 0 0 0 0.056248 0.056248 0.056248 0.056248
  spline S33 degree 5 poles (28.0734, 16.1624) (28.0438, 15.2899) (28.0325, 13.8524) (28.0901, 12.5348) (28.2108, 11.3251) (28.3896, 10.2086) (28.475, 9.7541) knots 0 0 0 0 0 0 0.2 0.345499 0.345499 0.345499 0.345499 0.345499 0.345499
  spline S34 degree 3 poles (3.3605, 43.321) (4.2972, 43.7123) (5.127, 43.7031) (6.3837, 43.2874) knots 0 0 0 0 1 1 1 1
  spline S35 degree 3 poles (6.3837, 43.2874) (7.3845, 42.9564) (8.1509, 42.4223) (9.1149, 41.384) knots 0 0 0 0 1 1 1 1
  spline S36 degree 3 poles (9.1149, 41.384) (9.6604, 40.7965) (9.9744, 40.5375) (10.1414, 40.5375) knots 0 0 0 0 1 1 1 1
  spline S37 degree 3 poles (10.1414, 40.5375) (10.2736, 40.5375) (10.8079, 40.801) (11.3285, 41.1231) knots 0 0 0 0 1 1 1 1
  spline S38 degree 3 poles (11.3285, 41.1231) (12.8148, 42.0424) (13.5925, 42.3956) (14.4099, 42.5224) knots 0 0 0 0 1 1 1 1
  spline S39 degree 3 poles (14.4099, 42.5224) (15.7434, 42.7294) (16.8719, 42.2963) (17.2889, 41.4175) knots 0 0 0 0 1 1 1 1
  spline S40 degree 3 poles (17.2889, 41.4175) (17.4425, 41.0937) (17.464, 40.8751) (17.4081, 40.2046) knots 0 0 0 0 1 1 1 1
  spline S41 degree 3 poles (17.4081, 40.2046) (17.3434, 39.4284) (17.3531, 39.3735) (17.5983, 39.1282) knots 0 0 0 0 1 1 1 1
  spline S42 degree 3 poles (17.5983, 39.1282) (17.8995, 38.827) (18.0838, 38.8152) (19.1861, 39.0261) knots 0 0 0 0 1 1 1 1
  spline S43 degree 3 poles (19.1861, 39.0261) (21.2987, 39.4304) (22.4511, 38.9297) (22.4522, 37.607) knots 0 0 0 0 1 1 1 1
  spline S44 degree 3 poles (22.4522, 37.607) (22.4529, 36.7454) (21.8377, 36.2639) (20.7361, 36.2639) knots 0 0 0 0 1 1 1 1
  spline S45 degree 3 poles (20.7361, 36.2639) (20.0382, 36.2639) (19.7425, 36.0347) (19.7425, 35.4937) knots 0 0 0 0 1 1 1 1
  spline S46 degree 3 poles (19.7425, 35.4937) (19.7425, 34.9001) (19.9962, 34.7075) (21.0588, 34.4943) knots 0 0 0 0 1 1 1 1
  spline S47 degree 3 poles (21.0588, 34.4943) (22.1331, 34.2788) (22.5478, 34.0955) (22.8603, 33.6982) knots 0 0 0 0 1 1 1 1
  spline S48 degree 3 poles (22.8603, 33.6982) (23.5958, 32.7632) (22.5543, 31.8861) (20.7083, 31.8861) knots 0 0 0 0 1 1 1 1
  spline S49 degree 3 poles (20.7083, 31.8861) (18.9346, 31.8861) (17.432, 32.5128) (15.9552, 33.8684) knots 0 0 0 0 1 1 1 1
  spline S50 degree 3 poles (15.9552, 33.8684) (15.4567, 34.326) (14.9608, 34.7004) (14.8533, 34.7004) knots 0 0 0 0 1 1 1 1
  spline S51 degree 3 poles (14.8533, 34.7004) (14.7458, 34.7004) (14.4299, 34.5351) (14.1513, 34.333) knots 0 0 0 0 1 1 1 1
  spline S52 degree 3 poles (14.1513, 34.333) (13.8727, 34.1309) (13.3868, 33.8381) (13.0715, 33.6822) knots 0 0 0 0 1 1 1 1
  spline S53 degree 3 poles (13.0715, 33.6822) (11.8711, 33.0889) (10.2509, 33.3985) (9.352, 34.393) knots 0 0 0 0 1 1 1 1
  spline S54 degree 3 poles (9.352, 34.393) (8.4004, 35.4459) (8.1864, 35.6385) (7.9683, 35.6385) knots 0 0 0 0 1 1 1 1
  spline S55 degree 3 poles (7.9683, 35.6385) (7.7171, 35.6385) (7.2977, 35.2383) (6.9738, 34.6891) knots 0 0 0 0 1 1 1 1
  spline S56 degree 3 poles (6.9738, 34.6891) (6.4989, 33.8843) (4.3788, 33.6094) (3.2207, 34.2025) knots 0 0 0 0 1 1 1 1
  spline S57 degree 3 poles (3.2207, 34.2025) (1.9483, 34.8542) (1.3752, 36.0623) (1.9202, 36.9441) knots 0 0 0 0 1 1 1 1
  spline S58 degree 3 poles (1.9202, 36.9441) (2.1572, 37.3277) (2.6853, 37.619) (3.1435, 37.619) knots 0 0 0 0 1 1 1 1
  spline S59 degree 3 poles (3.1435, 37.619) (3.8871, 37.619) (4.3159, 37.943) (4.3159, 38.505) knots 0 0 0 0 1 1 1 1
  spline S60 degree 3 poles (4.3159, 38.505) (4.3159, 39.0685) (4.1681, 39.1932) (3.1927, 39.4522) knots 0 0 0 0 1 1 1 1
  spline S61 degree 3 poles (3.1927, 39.4522) (2.8902, 39.5325) (2.529, 39.6727) (2.39, 39.7638) knots 0 0 0 0 1 1 1 1
  spline S62 degree 3 poles (2.39, 39.7638) (2.0795, 39.9672) (1.7097, 40.7046) (1.7111, 41.1177) knots 0 0 0 0 1 1 1 1
  spline S63 degree 3 poles (1.7111, 41.1177) (1.7137, 41.8847) (2.5286, 42.9734) (3.3605, 43.321) knots 0 0 0 0 1 1 1 1
  spline S64 degree 3 poles (40.3105, 43.3948) (41.3954, 43.901) (42.2636, 43.9539) (43.1464, 43.5675) knots 0 0 0 0 1 1 1 1
  spline S65 degree 3 poles (43.1464, 43.5675) (43.6121, 43.3637) (44.0986, 42.8484) (44.1975, 42.454) knots 0 0 0 0 1 1 1 1
  spline S66 degree 3 poles (44.1975, 42.454) (44.2329, 42.313) (44.2296, 41.9062) (44.1901, 41.55) knots 0 0 0 0 1 1 1 1
  spline S67 degree 3 poles (44.1901, 41.55) (44.0616, 40.3913) (44.0787, 40.2083) (44.3356, 40.0003) knots 0 0 0 0 1 1 1 1
  spline S68 degree 3 poles (44.3356, 40.0003) (44.7112, 39.6961) (45.1086, 39.7683) (46.0893, 40.3188) knots 0 0 0 0 1 1 1 1
  spline S69 degree 3 poles (46.0893, 40.3188) (47.5056, 41.1136) (48.2545, 41.3947) (49.1098, 41.4522) knots 0 0 0 0 1 1 1 1
  spline S70 degree 3 poles (49.1098, 41.4522) (50.0601, 41.5161) (50.6688, 41.3509) (51.2194, 40.8796) knots 0 0 0 0 1 1 1 1
  spline S71 degree 3 poles (51.2194, 40.8796) (51.7463, 40.4286) (51.9622, 40.0221) (51.9699, 39.4669) knots 0 0 0 0 1 1 1 1
  spline S72 degree 3 poles (51.9699, 39.4669) (51.9747, 39.1179) (51.9177, 38.9851) (51.6667, 38.7609) knots 0 0 0 0 1 1 1 1
  spline S73 degree 3 poles (51.6667, 38.7609) (51.4967, 38.6089) (51.1707, 38.4548) (50.9423, 38.4183) knots 0 0 0 0 1 1 1 1
  spline S74 degree 3 poles (50.9423, 38.4183) (50.0539, 38.2762) (49.4995, 37.6121) (49.7804, 37.0264) knots 0 0 0 0 1 1 1 1
  spline S75 degree 3 poles (49.7804, 37.0264) (49.9949, 36.579) (50.335, 36.453) (51.1465, 36.5202) knots 0 0 0 0 1 1 1 1
  spline S76 degree 3 poles (51.1465, 36.5202) (51.7992, 36.5743) (51.8736, 36.5589) (52.1107, 36.3219) knots 0 0 0 0 1 1 1 1
  spline S77 degree 3 poles (52.1107, 36.3219) (52.632, 35.8005) (52.3398, 34.5008) (51.5692, 33.913) knots 0 0 0 0 1 1 1 1
  spline S78 degree 3 poles (51.5692, 33.913) (50.1664, 32.8431) (48.1142, 32.4761) (46.4453, 32.9969) knots 0 0 0 0 1 1 1 1
  spline S79 degree 3 poles (46.4453, 32.9969) (45.8057, 33.1965) (44.9544, 33.904) (44.6602, 34.4802) knots 0 0 0 0 1 1 1 1
  spline S80 degree 3 poles (44.6602, 34.4802) (44.2129, 35.3568) (43.7112, 35.4679) (42.8564, 34.8799) knots 0 0 0 0 1 1 1 1
  spline S81 degree 3 poles (42.8564, 34.8799) (42.5554, 34.6729) (42.0276, 34.3719) (41.6837, 34.2111) knots 0 0 0 0 1 1 1 1
  spline S82 degree 3 poles (41.6837, 34.2111) (41.1075, 33.9417) (40.9598, 33.9187) (39.8075, 33.9187) knots 0 0 0 0 1 1 1 1
  line L8 (39.8075, 33.9187) -> (38.5567, 33.9187)
  line L9 (38.5567, 33.9187) -> (37.6186, 34.4148)
  spline S83 degree 3 poles (37.6186, 34.4148) (37.1026, 34.6877) (36.539, 34.9376) (36.3661, 34.9702) knots 0 0 0 0 1 1 1 1
  spline S84 degree 3 poles (36.3661, 34.9702) (35.922, 35.0539) (35.5337, 34.7143) (35.1462, 33.9031) knots 0 0 0 0 1 1 1 1
  spline S85 degree 3 poles (35.1462, 33.9031) (34.2767, 32.0829) (32.5077, 31.1785) (31.2082, 31.8899) knots 0 0 0 0 1 1 1 1
  spline S86 degree 3 poles (31.2082, 31.8899) (30.5745, 32.2368) (30.2974, 32.7818) (30.4669, 33.3475) knots 0 0 0 0 1 1 1 1
  spline S87 degree 3 poles (30.4669, 33.3475) (30.6161, 33.8457) (31.3598, 34.532) (32.2646, 35.0067) knots 0 0 0 0 1 1 1 1
  spline S88 degree 3 poles (32.2646, 35.0067) (33.1402, 35.466) (33.3971, 35.7096) (33.3971, 36.0805) knots 0 0 0 0 1 1 1 1
  spline S89 degree 3 poles (33.3971, 36.0805) (33.3971, 36.501) (33.238, 36.7542) (32.8468, 36.9565) knots 0 0 0 0 1 1 1 1
  spline S90 degree 3 poles (32.8468, 36.9565) (31.0444, 37.8883) (30.5759, 39.9699) (31.8443, 41.4109) knots 0 0 0 0 1 1 1 1
  spline S91 degree 3 poles (31.8443, 41.4109) (32.3815, 42.0212) (32.9483, 42.3169) (33.7139, 42.3863) knots 0 0 0 0 1 1 1 1
  spline S92 degree 3 poles (33.7139, 42.3863) (34.5937, 42.4661) (35.2523, 42.2098) (36.037, 41.4824) knots 0 0 0 0 1 1 1 1
  spline S93 degree 3 poles (36.037, 41.4824) (36.3909, 41.1543) (36.763, 40.8557) (36.8638, 40.8189) knots 0 0 0 0 1 1 1 1
  spline S94 degree 3 poles (36.8638, 40.8189) (37.192, 40.6989) (37.5089, 40.9167) (38.6147, 42.0227) knots 0 0 0 0 1 1 1 1
  spline S95 degree 3 poles (38.6147, 42.0227) (39.4081, 42.8162) (39.8679, 43.1882) (40.3105, 43.3948) knots 0 0 0 0 1 1 1 1
  spline S96 degree 3 poles (3.8396, 28.1591) (3.6928, 25.8896) (3.7601, 22.8302) (4.0082, 20.7539) knots 0 0 0 0 1 1 1 1
  ellipse E0 centre (58.4946, 46.0269) end of major axis (108.5558, 82.8636) minor radius 37.1858 (4.0082, 20.7539) -> (11.1287, 6.1499) ccw
  spline S97 degree 3 poles (11.1287, 6.1499) (15.8219, 1.7292) (21.8181, -0.6374) (28.7719, -0.8627) knots 0 0 0 0 1 1 1 1
  ellipse E1 centre (5.0131, 40.0097) end of major axis (43.6862, 4.3261) minor radius 27.1643 (28.7719, -0.8627) -> (39.0808, 0.9877) ccw
  spline S98 degree 3 poles (39.0808, 0.9877) (40.5743, 1.6901) (41.6727, 2.4153) (42.7258, 3.4112) knots 0 0 0 0 1 1 1 1
  spline S99 degree 3 poles (42.7258, 3.4112) (44.4016, 4.9959) (45.589, 6.8874) (46.5056, 9.5421) (46.9414, 10.8042) (47.3249, 12.2429) (47.6965, 13.9335) knots 0 0 0 0 0.677783 0.677783 0.677783 1 1 1 1
  spline S100 degree 3 poles (47.6965, 13.9335) (48.7263, 18.6186) (49.1132, 21.8227) (49.3958, 27.9744) knots 0 0 0 0 1 1 1 1
  ellipse E2 centre (49.445, 28.2243) end of major axis (49.5599, 30.6408) minor radius 0.0375 (49.4993, 29.9265) -> (49.3958, 27.9744) ccw
  spline S101 degree 3 poles (49.4993, 29.9265) (51.3935, 30.3328) (52.9435, 31.0564) (54.0116, 32.193) (54.363, 32.5669) (54.6579, 32.9856) (54.882, 33.4409) knots 0.033409 0.033409 0.033409 0.033409 0.760746 0.760746 0.760746 0.999997 0.999997 0.999997 0.999997
  spline S102 degree 3 poles (54.882, 33.4409) (55.0347, 33.7513) (55.1727, 34.0995) (55.2323, 34.4752) (55.2709, 34.7187) (55.2821, 34.9498) (55.2846, 35.2136) knots 0 0 0 0 0.549059 0.549059 0.549059 0.90483 0.90483 0.90483 0.90483
  line L10 (55.2846, 35.2136) -> (55.2832, 35.6451)
  spline S103 degree 3 poles (55.2832, 35.6451) (55.2771, 35.9972) (55.2543, 36.309) (55.1786, 36.6345) (55.1024, 36.9617) (54.9878, 37.2507) (54.8436, 37.5871) knots 0.088946 0.088946 0.088946 0.088946 0.543269 0.543269 0.543269 1 1 1 1
  line L11 (54.8436, 37.5871) -> (54.6708, 37.9902)
  line L12 (54.6708, 37.9902) -> (54.7256, 38.1789)
  spline S104 degree 3 poles (54.7256, 38.1789) (55.1949, 39.793) (54.7298, 41.4712) (53.6604, 42.6498) (52.9721, 43.4084) (52.0402, 43.976) (50.9574, 44.2653) knots 0 0 0 0 0.608426 0.608426 0.608426 1 1 1 1
  spline S105 degree 3 poles (50.9574, 44.2653) (49.8818, 44.5526) (48.7117, 44.4734) (47.3744, 44.1183) (47.178, 44.0661) (46.9771, 44.0079) (46.771, 43.9438) knots 0 0 0 0 0.824545 0.824545 0.824545 0.945665 0.945665 0.945665 0.945665
  spline S106 degree 3 poles (46.771, 43.9438) (46.7093, 44.062) (46.6405, 44.1796) (46.5676, 44.2944) (46.2623, 44.7749) (45.8902, 45.2321) (45.4363, 45.6075) (45.3884, 45.647) (45.3392, 45.6858) (45.2879, 45.7236) knots 0.223295 0.223295 0.223295 0.223295 0.361232 0.361232 0.361232 0.939053 0.939053 0.939053 1 1 1 1
  spline S107 degree 3 poles (45.2879, 45.7236) (44.2745, 46.4714) (42.9911, 46.772) (41.707, 46.737) (41.2318, 46.724) (40.7551, 46.6601) (40.2904, 46.5351) knots 0.000002 0.000002 0.000002 0.000002 0.729882 0.729882 0.729882 1 1 1 1
  spline S108 degree 3 poles (40.2904, 46.5351) (39.1403, 46.2258) (38.0053, 45.5417) (37.0282, 44.651) knots 0.000001 0.000001 0.000001 0.000001 1 1 1 1
  line L13 (37.0282, 44.651) -> (36.9035, 44.5374)
  spline S109 degree 3 poles (36.9035, 44.5374) (35.1678, 45.5188) (33.1775, 45.6076) (31.5191, 44.8193) (30.4628, 44.3172) (29.5504, 43.4745) (28.8905, 42.373) knots 0.019099 0.019099 0.019099 0.019099 0.618328 0.618328 0.618328 1 1 1 1
  spline S110 degree 3 poles (28.8905, 42.373) (28.2356, 41.2799) (28.0251, 39.987) (28.2891, 38.7134) (28.4327, 38.0204) (28.7011, 37.3303) (29.0737, 36.6286) knots 0 0 0 0 0.647645 0.647645 0.647645 1 1 1 1
  line L14 (29.0737, 36.6286) -> (29.1612, 36.4638)
  line L15 (29.1612, 36.4638) -> (28.9908, 36.2914)
  spline S111 degree 3 poles (28.9908, 36.2914) (28.3897, 35.6836) (27.931, 35.0843) (27.6841, 34.3672) (27.522, 33.8963) (27.4651, 33.4076) (27.4689, 32.9193) knots 0 0 0 0 0.603605 0.603605 0.603605 1 1 1 1
  spline S112 degree 3 poles (27.4689, 32.9193) (27.4781, 31.7149) (28.0681, 30.6219) (28.9533, 29.8689) (29.5522, 29.3594) (30.2878, 28.9905) (31.1058, 28.7908) knots 0 0 0 0 0.569109 0.569109 0.569109 0.954182 0.954182 0.954182 0.954182
  ellipse E3 centre (31.0764, 27.6801) end of major axis (31.0429, 29.675) minor radius 0.0578 (31.1352, 27.6181) -> (31.1058, 28.7908) ccw
  spline S113 degree 3 poles (31.1352, 27.6181) (31.1644, 25.7831) (31.0814, 24.7731) (30.8193, 23.7418) (30.754, 23.485) (30.6766, 23.2243) (30.5839, 22.9462) knots 0 0 0 0 0.800641 0.800641 0.800641 1 1 1 1
  spline S114 degree 3 poles (30.5839, 22.9462) (29.9756, 21.1214) (28.9014, 19.8352) (27.6291, 19.2047) knots 0 0 0 0 1 1 1 1
  spline S115 degree 3 poles (27.6291, 19.2047) (26.8945, 18.8407) (26.4461, 18.7298) (25.9454, 18.7349) (25.7421, 18.7369) (25.5228, 18.7611) (25.2651, 18.8137) knots 0 0 0 0 0.711303 0.711303 0.711303 1 1 1 1
  spline S116 degree 3 poles (25.2651, 18.8137) (23.7232, 19.1281) (22.4595, 20.0877) (21.5265, 21.709) (21.0344, 22.5641) (20.647, 23.6026) (20.4034, 24.8024) knots 0 0 0 0 0.654705 0.654705 0.654705 1 1 1 1
  spline S117 degree 3 poles (20.4034, 24.8024) (20.2739, 25.4408) (20.1421, 26.5799) (20.0696, 27.6039) (20.0342, 28.1041) (20.0114, 28.5828) (20.0045, 28.9687) knots 0 0 0 0 0.457255 0.457255 0.457255 0.680586 0.680586 0.680586 0.680586
  ellipse E4 centre (21.8994, 28.801) end of major axis (24.7102, 28.7135) minor radius 0.1473 (20.5728, 28.9721) -> (20.0045, 28.9687) ccw
  spline S118 degree 3 poles (20.5728, 28.9721) (21.4581, 28.9695) (21.9205, 28.9661) (22.3941, 29.0471) (22.71, 29.1012) (22.9935, 29.2034) (23.2325, 29.3044) knots 0 0 0 0 0.599835 0.599835 0.599835 1 1 1 1
  spline S119 degree 3 poles (23.2325, 29.3044) (24.2399, 29.7303) (25.0756, 30.3613) (25.5649, 31.2416) (25.8255, 31.7103) (25.9766, 32.236) (26.0196, 32.7724) knots 0.000002 0.000002 0.000002 0.000002 0.65253 0.65253 0.65253 1 1 1 1
  spline S120 degree 3 poles (26.0196, 32.7724) (26.0464, 33.1056) (26.0575, 33.4303) (25.9898, 33.7774) (25.9304, 34.0819) (25.8237, 34.343) (25.7057, 34.6008) knots 0 0 0 0 0.532706 0.532706 0.532706 1 1 1 1
  ellipse E5 centre (16.0287, 33.8196) end of major axis (26.0555, 32.469) minor radius 5.942 (25.7057, 34.6008) -> (25.0063, 35.7274) ccw
  spline S121 degree 3 poles (25.0063, 35.7274) (25.2152, 36.1653) (25.3445, 36.6528) (25.3876, 37.161) (25.3966, 37.268) (25.4033, 37.3773) (25.4085, 37.4918) knots 0.077995 0.077995 0.077995 0.077995 0.83962 0.83962 0.83962 1 1 1 1
  spline S122 degree 3 poles (25.4085, 37.4918) (25.4258, 37.868) (25.439, 38.1756) (25.3733, 38.5347) (25.3129, 38.8652) (25.1915, 39.151) (25.0593, 39.4265) (25.0387, 39.4695) (25.0174, 39.513) (24.9954, 39.5579) knots 0 0 0 0 0.484601 0.484601 0.484601 0.930484 0.930484 0.930484 1 1 1 1
  spline S123 degree 3 poles (24.9954, 39.5579) (24.5918, 40.3776) (23.9772, 41.085) (23.1648, 41.5103) (22.385, 41.9186) (21.4967, 42.0784) (20.4603, 42.1269) knots 0 0 0 0 0.510228 0.510228 0.510228 1 1 1 1
  line L16 (20.4603, 42.1269) -> (20.1789, 42.1401)